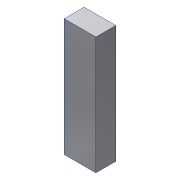
# Autodesk Inventor part: Distanzblock
Saved by Autodesk Inventor 2016 (Build 200138000, 138)
## iProperties
Created: 2015-07-27
Part Number: Distanzblock
Material: Aluminum 6061
Document SubType Name: Modeling
Density: 2.7 g/cm^3
Appearance: Aluminum - Flat
Autodesk Inventor part; units mm, degrees
ref_plane "YZ Plane" through (0, 0, 0) normal (1, 0, 0) x (0, 1, 0)
ref_plane "XZ Plane" through (0, 0, 0) normal (0, 1, 0) x (-1, 0, 0)
ref_plane "XY Plane" through (0, 0, 0) normal (0, 0, 1) x (1, 0, 0)
sketch "Sketch1" plane through (0, 0, 0) normal (0, 0, 1) x (1, 0, 0)
  line L0 (-17.5, -11) -> (17.5, -11)
  line L1 (17.5, -11) -> (17.5, 11)
  line L2 (17.5, 11) -> (-17.5, 11)
  line L3 (-17.5, 11) -> (-17.5, -11)
  line L4 (-17.5, -11) -> (17.5, 11) construction
  line L5 (17.5, -11) -> (-17.5, 11) construction
  point P0 (0, 0)
  dimension "d0" = 35
  dimension "d1" = 22
  constraints: 12 end point, 2 midpoint, 2 parallel, 1 horizontal, 1 perpendicular
  measures "d0" distance of L2.end L1.end
  measures "d1" distance of L1.end L0.end
extrude "Extrusion1" add sketch "Sketch1" along normal blind 130
body "Solid1"
